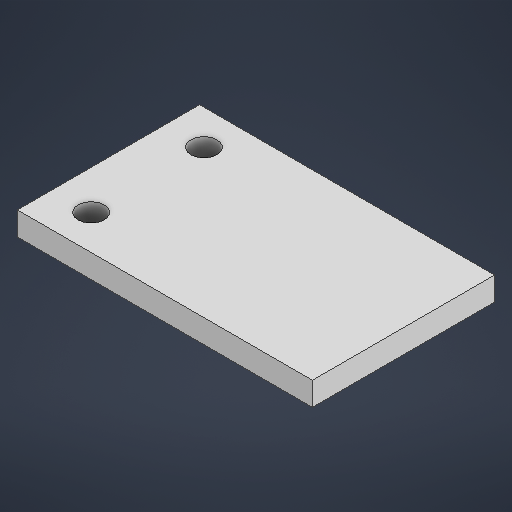
# Autodesk Inventor part: Scheda cella di carico
Saved by Autodesk Inventor 2026.2 (Build 302298000, 298)
## iProperties
Created: 2026-01-19
Part Number: Scheda cella di carico
Material: Generic
Document SubType Name: Modeling
Designer: ASUS
Density: 1 g/cm^3
Appearance: Default
Author: ASUS
Autodesk Inventor part; units mm, degrees
ref_plane "YZ Plane" through (0, 0, 0) normal (1, 0, 0) x (0, 1, 0)
ref_plane "XZ Plane" through (0, 0, 0) normal (0, 1, 0) x (-1, 0, 0)
ref_plane "XY Plane" through (0, 0, 0) normal (0, 0, 1) x (1, 0, 0)
sketch "Sketch1" plane through (0, 0, 0) normal (0, 1, 0) x (-1, 0, 0)
  line L0 (0, 0) -> (-34, 0)
  line L1 (-34, 0) -> (-34, -21)
  line L2 (-34, -21) -> (0, -21)
  line L3 (0, -21) -> (0, 0)
  dimension "d0" = 34
  dimension "d1" = 21
  constraints: 8 end point, 2 parallel, 1 horizontal, 1 perpendicular
  measures "d0" distance of L2.end L1.end
  measures "d1" distance of L1.end L0.end
extrude "Extrusion1" add sketch "Sketch1" along normal blind 2.7
sketch "Sketch2" plane through (0, 0, 0) normal (0, -1, 0) x (1, 0, 0)
  line L0 (0, 0) -> (4.5, 0)
  line L1 (0, 0) -> (34, 0) projected
  circle A0 centre (4.5, -4) radius 1.5
  line L2 (34, 0) -> (34, -21) projected
  line L3 (0, -21) -> (0, 0) projected
  circle A1 centre (4.5, -17) radius 1.5
  dimension "d4" = 4.5
  dimension "d6" = 3
  constraints: 2 centre point, 2 end point, 1 point on line
  measures "d4" distance of L0.start L0.end
  measures "d6" diameter of A0
extrude "Extrusion2" cut sketch "Sketch2" against normal blind 2.7
body "Solid1"
